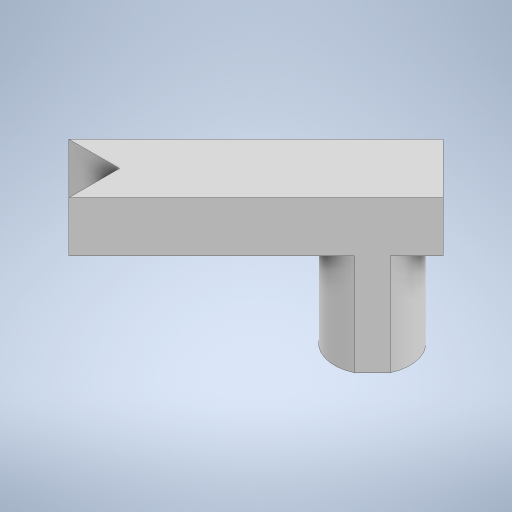
# Autodesk Inventor part: hjørner holder
Saved by Autodesk Inventor 2024 (Build 280153000, 153)
## iProperties
Created: 2024-03-15
Part Number: hjørner holder
Material: Generic
Document SubType Name: Modeling
Designer: laura
Density: 1 g/cm^3
Appearance: Default
Author: laura
Autodesk Inventor part; units mm, degrees
ref_plane "YZ Plane" through (0, 0, 0) normal (1, 0, 0) x (0, 1, 0)
ref_plane "XZ Plane" through (0, 0, 0) normal (0, 1, 0) x (-1, 0, 0)
ref_plane "XY Plane" through (0, 0, 0) normal (0, 0, 1) x (1, 0, 0)
sketch "Sketch1" plane through (0, 0, 0) normal (0, 1, 0) x (-1, 0, 0)
  circle A0 centre (25, -25) radius 7.5
  line L0 (50, 0) -> (60, 0)
  line L1 (50, 10) -> (50, 0)
  line L2 (60, 0) -> (22.9954, -37.0046)
  line L3 (60, 0) -> (112.3325, 0) construction
  line L4 (50, 10) -> (12.9954, -27.0046)
  line L5 (50, 10) -> (102.3325, 10) construction
  line L6 (12.9954, -27.0046) -> (22.9954, -37.0046)
  point P0 (0, 0)
  point P1 (21.7678, -18.2322)
  point P2 (18.2322, -21.7678)
  point P3 (28.2322, -31.7678)
  point P4 (31.7678, -28.2322)
  dimension "d2" = 15
  dimension "d7" = 135
  dimension "d8" = 135
  constraints: 14 end point, 3 horizontal, 2 equal length, 1 centre point, 1 perpendicular
  measures "d2" diameter of A0
  measures "d7" angle of L2 L3
  measures "d8" angle of L4 L5
extrude "Extrusion1" add sketch "Sketch1" along normal blind 10 contours A0 L2 L4 | A0 L4 L1 L0 L2 | A0 L2 L6 L4
extrude "Extrusion2" add sketch "Sketch1" against normal blind 20 contours A0 L2 L4
body "Solid1"
